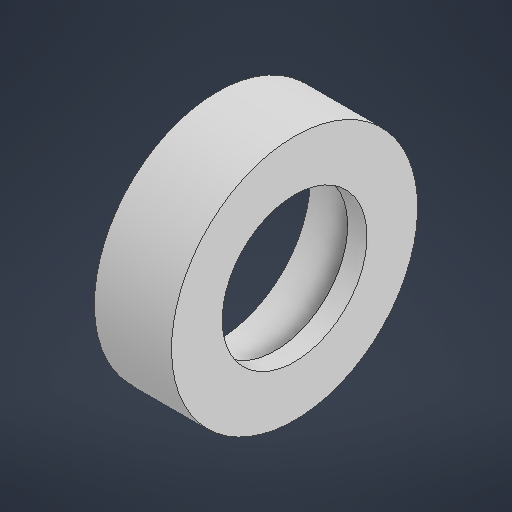
# Autodesk Inventor part: P_Lagerschale
Saved by Autodesk Inventor 2026 (Build 300175000, 175)
## iProperties
Created: 2025-04-25
Part Number: P_Lagerschale
Material: Generisch
Document SubType Name: Modeling
Designer: FAL
Density: 1 g/cm^3
Appearance: Vorgabe
Author: FAL
Autodesk Inventor part; units mm, degrees
ref_plane "YZ Plane" through (0, 0, 0) normal (1, 0, 0) x (0, 1, 0)
ref_plane "XZ Plane" through (0, 0, 0) normal (0, 1, 0) x (-1, 0, 0)
ref_plane "XY Plane" through (0, 0, 0) normal (0, 0, 1) x (1, 0, 0)
sketch "Skizze1" plane through (0, 0, 0) normal (0, 1, 0) x (-1, 0, 0)
  line L0 (0, 0) -> (27.8247, 0)
  line L1 (0, 7.5) -> (0, 12.75)
  line L2 (0, 12.75) -> (8, 12.75)
  line L3 (8, 12.75) -> (8, 9.6)
  line L4 (8, 9.6) -> (2, 9.6)
  line L5 (2, 9.6) -> (2, 7.5)
  line L6 (2, 7.5) -> (0, 7.5)
  line L7 (0, 7.5) -> (0, 0) construction
  point P0 (5, 9.6)
  dimension "d0" = 25.5
  dimension "d1" = 15
  dimension "d2" = 19.2
  dimension "d3" = 6
  dimension "d4" = 2
  constraints: 16 end point, 6 perpendicular, 2 point on line, 1 collinear, 1 horizontal, 1 midpoint, 1 vertical
  measures "d0" diameter of L2 L0
  measures "d1" diameter of L6 L0
  measures "d2" diameter of point (5, 9.6) L0
  measures "d3" distance between parallel lines of L3 L5
  measures "d4" distance between parallel lines of L5 L1
revolve "Umdrehung1" add sketch "Skizze1" angle 360 about axis through (0, 0, 0) along (-1, 0, 0)
sketch "Skizze2" plane through (-8, 0, 0) normal (-1, 0, 0) x (0, 0, 1)
  point P0 (0, 0)
sketch "Skizze3" plane through (-8, 0, 0) normal (-1, 0, 0) x (0, 0, 1)
  circle A0 centre (0, 0) radius 12.75 projected
  line L0 (0, 12.75) -> (0, 9.6) construction
  circle A1 centre (0, 0) radius 9.6 projected
  circle A2 centre (0, 11.175) radius 0.95
  dimension "d6" = 1.9
  constraints: 2 end point, 2 vertical alignment, 1 centre point, 1 midpoint, 1 vertical, 2 other
  measures "d6" diameter of A2
extrude "Extrusion1" cut sketch "Skizze3" against normal blind 4 contours A2
pattern_circular "Runde Anordnung1" count 3 over 360 about axis through (-5, 0, 0) along (-1, 0, 0) of "Extrusion1"
